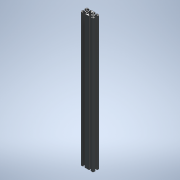
# Autodesk Inventor part: Profil_40x20_500
Saved by Autodesk Inventor 2022 (Build 260153000, 153)
## iProperties
Created: 2021-11-30
Part Number: Profil_40x20_500
Material: Generic
Document SubType Name: Modeling
Designer: Fabijan_Sven
Density: 1 g/cm^3
Appearance: Default
Author: Fabijan_Sven
Autodesk Inventor part; units mm, degrees
ref_plane "YZ Plane" through (0, 0, 0) normal (1, 0, 0) x (0, 1, 0)
ref_plane "XZ Plane" through (0, 0, 0) normal (0, 1, 0) x (-1, 0, 0)
ref_plane "XY Plane" through (0, 0, 0) normal (0, 0, 1) x (1, 0, 0)
sketch "Sketch1" plane through (0, 0, 0) normal (0, 1, 0) x (-1, 0, 0)
  line L0 (8, 10) -> (3, 10)
  line L1 (10, 3) -> (10, 8)
  line L2 (2.5, 9.5) -> (2.5, 8.2)
  line L3 (2.5, 8.2) -> (5.7198, 8.2)
  line L4 (6.0734, 7.3464) -> (3.2627, 4.5358)
  line L5 (1.8485, 3.95) -> (0, 3.95)
  line L6 (0, 3.95) -> (0, 2.15)
  line L7 (0, 2.15) -> (0, 2.15)
  line L8 (2.15, 0) -> (2.15, 0)
  line L9 (2.15, 0) -> (3.95, 0)
  line L10 (8.2, 5.7204) -> (8.2, 2.5)
  line L11 (8.2, 2.5) -> (9.5, 2.5)
  line L12 (0, 29.0836) -> (0, -4.1523) construction
  line L13 (3.95, 0) -> (3.95, 1.8491)
  line L14 (7.3464, 6.0739) -> (4.5358, 3.2633)
  arc A0 (10, 8) -> (8, 10) centre (8, 8) ccw
  arc A1 (8.2, 5.7204) -> (7.3464, 6.0739) centre (7.7, 5.7204) ccw
  arc A2 (6.0734, 7.3464) -> (5.7198, 8.2) centre (5.7198, 7.7) ccw
  arc A3 (4.5358, 3.2633) -> (3.95, 1.8491) centre (5.95, 1.8491) ccw
  arc A4 (1.8485, 3.95) -> (3.2627, 4.5358) centre (1.8485, 5.95) ccw
  arc A5 (2.15, 0) -> (0, 2.15) centre (0, 0) ccw
  arc A6 (3, 10) -> (2.5, 9.5) centre (3, 9.5) ccw
  arc A7 (9.5, 2.5) -> (10, 3) centre (9.5, 3) ccw
  line L15 (18.5462, 0) -> (-9.9601, 0) construction
  line L16 (-3, 10) -> (-8, 10)
  arc A8 (-2.5, 9.5) -> (-3, 10) centre (-3, 9.5) ccw
  line L17 (-2.5, 8.2) -> (-2.5, 9.5)
  line L18 (-5.7204, 8.2) -> (-2.5, 8.2)
  arc A9 (-5.7204, 8.2) -> (-6.0739, 7.3464) centre (-5.7204, 7.7) ccw
  line L19 (-6.0739, 7.3464) -> (-3.2633, 4.5358)
  arc A10 (-3.2633, 4.5358) -> (-1.8491, 3.95) centre (-1.8491, 5.95) ccw
  line L20 (0, 3.95) -> (-1.8491, 3.95)
  line L21 (0, 2.15) -> (0, 3.95)
  arc A11 (0, 2.15) -> (-2.15, 0) centre (0, 0) ccw
  line L22 (-3.95, 0) -> (-2.15, 0)
  line L23 (-3.95, 1.8485) -> (-3.95, 0)
  arc A12 (-3.95, 1.8485) -> (-4.5358, 3.2627) centre (-5.95, 1.8485) ccw
  line L24 (-7.3464, 6.0734) -> (-4.5358, 3.2627)
  arc A13 (-7.3464, 6.0734) -> (-8.2, 5.7198) centre (-7.7, 5.7198) ccw
  line L25 (-8.2, 2.5) -> (-8.2, 5.7198)
  line L26 (-9.5, 2.5) -> (-8.2, 2.5)
  arc A14 (-10, 3) -> (-9.5, 2.5) centre (-9.5, 3) ccw
  line L27 (-10, 8) -> (-10, 3)
  arc A15 (-8, 10) -> (-10, 8) centre (-8, 8) ccw
  line L28 (-10, -3) -> (-10, -8)
  arc A16 (-9.5, -2.5) -> (-10, -3) centre (-9.5, -3) ccw
  line L29 (-8.2, -2.5) -> (-9.5, -2.5)
  line L30 (-8.2, -5.7204) -> (-8.2, -2.5)
  arc A17 (-8.2, -5.7204) -> (-7.3464, -6.0739) centre (-7.7, -5.7204) ccw
  line L31 (-7.3464, -6.0739) -> (-4.5358, -3.2633)
  arc A18 (-4.5358, -3.2633) -> (-3.95, -1.8491) centre (-5.95, -1.8491) ccw
  line L32 (-3.95, 0) -> (-3.95, -1.8491)
  line L33 (-2.15, 0) -> (-3.95, 0)
  arc A19 (-2.15, 0) -> (0, -2.15) centre (0, 0) ccw
  line L34 (0, -3.95) -> (0, -2.15)
  line L35 (-1.8485, -3.95) -> (0, -3.95)
  arc A20 (-1.8485, -3.95) -> (-3.2627, -4.5358) centre (-1.8485, -5.95) ccw
  line L36 (-6.0734, -7.3464) -> (-3.2627, -4.5358)
  arc A21 (-6.0734, -7.3464) -> (-5.7198, -8.2) centre (-5.7198, -7.7) ccw
  line L37 (-2.5, -8.2) -> (-5.7198, -8.2)
  line L38 (-2.5, -9.5) -> (-2.5, -8.2)
  arc A22 (-3, -10) -> (-2.5, -9.5) centre (-3, -9.5) ccw
  line L39 (-8, -10) -> (-3, -10)
  arc A23 (-10, -8) -> (-8, -10) centre (-8, -8) ccw
  line L40 (3, -10) -> (8, -10)
  arc A24 (2.5, -9.5) -> (3, -10) centre (3, -9.5) ccw
  line L41 (2.5, -8.2) -> (2.5, -9.5)
  line L42 (5.7204, -8.2) -> (2.5, -8.2)
  arc A25 (5.7204, -8.2) -> (6.0739, -7.3464) centre (5.7204, -7.7) ccw
  line L43 (6.0739, -7.3464) -> (3.2633, -4.5358)
  arc A26 (3.2633, -4.5358) -> (1.8491, -3.95) centre (1.8491, -5.95) ccw
  line L44 (0, -3.95) -> (1.8491, -3.95)
  line L45 (0, -2.15) -> (0, -3.95)
  arc A27 (0, -2.15) -> (2.15, 0) centre (0, 0) ccw
  line L46 (3.95, 0) -> (2.15, 0)
  line L47 (3.95, -1.8485) -> (3.95, 0)
  arc A28 (3.95, -1.8485) -> (4.5358, -3.2627) centre (5.95, -1.8485) ccw
  line L48 (7.3464, -6.0734) -> (4.5358, -3.2627)
  arc A29 (7.3464, -6.0734) -> (8.2, -5.7198) centre (7.7, -5.7198) ccw
  line L49 (8.2, -2.5) -> (8.2, -5.7198)
  line L50 (9.5, -2.5) -> (8.2, -2.5)
  arc A30 (10, -3) -> (9.5, -2.5) centre (9.5, -3) ccw
  line L51 (10, -8) -> (10, -3)
  arc A31 (8, -10) -> (10, -8) centre (8, -8) ccw
  line L52 (-25.7204, 8.2) -> (-22.5, 8.2)
  line L53 (-22.5, 8.2) -> (-22.5, 9.5)
  arc A32 (-22.5, 9.5) -> (-23, 10) centre (-23, 9.5) ccw
  line L54 (-23, 10) -> (-28, 10)
  line L55 (-18.1515, 3.95) -> (-20, 3.95)
  line L56 (-20, 2.15) -> (-20, 2.15)
  line L57 (-17.85, 0) -> (-17.85, 0)
  line L58 (-17.85, 0) -> (-16.05, 0)
  line L59 (-11.8, 2.5) -> (-10.5, 2.5)
  line L60 (-1.4538, 0) -> (-29.9601, 0) construction
  line L61 (-16.05, 0) -> (-16.05, 1.8491)
  arc A33 (-15.4642, 3.2633) -> (-16.05, 1.8491) centre (-14.05, 1.8491) ccw
  arc A34 (-17.85, 0) -> (-20, 2.15) centre (-20, 0) ccw
  line L62 (-20, 3.95) -> (-20, 2.15)
  line L63 (-20, 3.95) -> (-21.8491, 3.95)
  arc A35 (-23.2633, 4.5358) -> (-21.8491, 3.95) centre (-21.8491, 5.95) ccw
  line L64 (-20, 2.15) -> (-20, 3.95)
  arc A36 (-20, 2.15) -> (-22.15, 0) centre (-20, 0) ccw
  arc A37 (-10.5, 2.5) -> (-10, 3) centre (-10.5, 3) ccw
  line L65 (-12.6536, -6.0734) -> (-15.4642, -3.2627)
  line L66 (-10.5, -2.5) -> (-11.8, -2.5)
  line L67 (-13.9261, -7.3464) -> (-16.7367, -4.5358)
  arc A38 (-10, -3) -> (-10.5, -2.5) centre (-10.5, -3) ccw
  line L68 (-14.2796, -8.2) -> (-17.5, -8.2)
  arc A39 (-12.6536, -6.0734) -> (-11.8, -5.7198) centre (-12.3, -5.7198) ccw
  arc A40 (-14.2796, -8.2) -> (-13.9261, -7.3464) centre (-14.2796, -7.7) ccw
  line L69 (-17, -10) -> (-12, -10)
  line L70 (-10, -8) -> (-10, -3)
  line L71 (-11.8, -2.5) -> (-11.8, -5.7198)
  arc A41 (-12, -10) -> (-10, -8) centre (-12, -8) ccw
  arc A42 (-25.7204, 8.2) -> (-26.0739, 7.3464) centre (-25.7204, 7.7) ccw
  arc A43 (-28, 10) -> (-30, 8) centre (-28, 8) ccw
  arc A44 (-27.3464, 6.0734) -> (-28.2, 5.7198) centre (-27.7, 5.7198) ccw
  line L72 (-26.0739, 7.3464) -> (-23.2633, 4.5358)
  line L73 (-27.3464, 6.0734) -> (-24.5358, 3.2627)
  arc A45 (-23.95, 1.8485) -> (-24.5358, 3.2627) centre (-25.95, 1.8485) ccw
  line L74 (-28.2, 2.5) -> (-28.2, 5.7198)
  line L75 (-30, 8) -> (-30, 3)
  line L76 (-29.5, 2.5) -> (-28.2, 2.5)
  arc A46 (-30, 3) -> (-29.5, 2.5) centre (-29.5, 3) ccw
  line L77 (-23.95, 0) -> (-22.15, 0)
  line L78 (-22.15, 0) -> (-23.95, 0)
  arc A47 (-22.15, 0) -> (-20, -2.15) centre (-20, 0) ccw
  line L79 (-23.95, 0) -> (-23.95, -1.8491)
  arc A48 (-24.5358, -3.2633) -> (-23.95, -1.8491) centre (-25.95, -1.8491) ccw
  line L80 (-21.8485, -3.95) -> (-20, -3.95)
  line L81 (-20, -3.95) -> (-20, -2.15)
  line L82 (-20, -2.15) -> (-20, -3.95)
  line L83 (-17.5, 9.5) -> (-17.5, 8.2)
  arc A49 (-18.1515, 3.95) -> (-16.7373, 4.5358) centre (-18.1515, 5.95) ccw
  arc A50 (-17, 10) -> (-17.5, 9.5) centre (-17, 9.5) ccw
  line L84 (-17.5, 8.2) -> (-14.2802, 8.2)
  line L85 (-13.9266, 7.3464) -> (-16.7373, 4.5358)
  arc A51 (-13.9266, 7.3464) -> (-14.2802, 8.2) centre (-14.2802, 7.7) ccw
  line L86 (-12.6536, 6.0739) -> (-15.4642, 3.2633)
  line L87 (-11.8, 5.7204) -> (-11.8, 2.5)
  arc A52 (-11.8, 5.7204) -> (-12.6536, 6.0739) centre (-12.3, 5.7204) ccw
  line L88 (-12, 10) -> (-17, 10)
  line L89 (-10, 3) -> (-10, 8)
  arc A53 (-10, 8) -> (-12, 10) centre (-12, 8) ccw
  line L90 (-30, -3) -> (-30, -8)
  arc A54 (-28.2, -5.7204) -> (-27.3464, -6.0739) centre (-27.7, -5.7204) ccw
  arc A55 (-30, -8) -> (-28, -10) centre (-28, -8) ccw
  line L91 (-27.3464, -6.0739) -> (-24.5358, -3.2633)
  arc A56 (-26.0734, -7.3464) -> (-25.7198, -8.2) centre (-25.7198, -7.7) ccw
  line L92 (-26.0734, -7.3464) -> (-23.2627, -4.5358)
  arc A57 (-21.8485, -3.95) -> (-23.2627, -4.5358) centre (-21.8485, -5.95) ccw
  line L93 (-28, -10) -> (-23, -10)
  line L94 (-22.5, -8.2) -> (-25.7198, -8.2)
  line L95 (-22.5, -9.5) -> (-22.5, -8.2)
  arc A58 (-23, -10) -> (-22.5, -9.5) centre (-23, -9.5) ccw
  line L96 (-20, -3.95) -> (-18.1509, -3.95)
  arc A59 (-20, -2.15) -> (-17.85, 0) centre (-20, 0) ccw
  line L97 (-16.05, -1.8485) -> (-16.05, 0)
  line L98 (-16.05, 0) -> (-17.85, 0)
  arc A60 (-16.05, -1.8485) -> (-15.4642, -3.2627) centre (-14.05, -1.8485) ccw
  arc A61 (-16.7367, -4.5358) -> (-18.1509, -3.95) centre (-18.1509, -5.95) ccw
  line L99 (-23.95, 1.8485) -> (-23.95, 0)
  line L100 (-17.5, -8.2) -> (-17.5, -9.5)
  arc A62 (-17.5, -9.5) -> (-17, -10) centre (-17, -9.5) ccw
  line L101 (-28.2, -5.7204) -> (-28.2, -2.5)
  line L102 (-28.2, -2.5) -> (-29.5, -2.5)
  arc A63 (-29.5, -2.5) -> (-30, -3) centre (-29.5, -3) ccw
  line L103 (-8, -10) -> (-12, -10)
  line L104 (-8, 10) -> (-12, 10)
  point P0 (0, 0)
  point P1 (3.95, 2.6775)
  point P2 (-2.6775, 3.95)
  point P3 (0, 0)
  point P4 (-3.95, -2.6775)
  point P5 (0, 0)
  point P6 (2.6775, -3.95)
  point P7 (0, 0)
  point P8 (-20, 0)
  point P9 (-16.05, 2.6775)
  point P10 (-20, -4.1523)
  point P11 (-22.6775, 3.95)
  point P12 (-20, 0)
  point P13 (-20, 0)
  point P14 (-20, 0)
  point P15 (-17.3225, -3.95)
  point P16 (-23.95, -2.6775)
  point P17 (-10, 3)
  dimension "d1" = 2.5
  dimension "d2" = 2.5
  dimension "d3" = 1.8
  dimension "d4" = 1.8
  dimension "d5" = 45
  dimension "d6" = 2.15
  dimension "d7" = 2.15
  dimension "d8" = 1.8
  dimension "d11" = 10
  dimension "d12" = 10
  dimension "d14" = 1.8
  dimension "d15" = 1.8
  dimension "d16" = 2.6775
  dimension "d18" = 2
  dimension "d19" = 0.5
  dimension "d20" = 2
  dimension "d21" = 2.15
  dimension "d22" = 0.5
  dimension "d25" = 360
  dimension "d31" = 20
  constraints: 210 end point, 128 point on circle, 64 centre point, 32 point on line, 16 tangent, 5 perpendicular, 5 vertical, 4 parallel, 3 equal radius, 3 horizontal, 2 coincident, 1 collinear, 420 other
  measures "d1" distance from line of point (0, 0) L2
  measures "d2" distance from line of point (0, 0) L11
  measures "d3" distance between parallel lines of L10 L1
  measures "d4" distance between parallel lines of L0 L3
  measures "d5" angle of L4 L12
  measures "d6" distance of point (0, 0) L6.end
  measures "d7" distance from line of point (0, 0) L8
  measures "d8" distance between parallel lines of L5 L7
  measures "d11" distance from line of point (0, 0) L0
  measures "d12" distance from line of point (0, 0) L1
  measures "d14" distance between parallel lines of L8 L13
  measures "d15" distance between parallel lines of L4 L14
  measures "d16" distance of L9.end point (3.95, 2.678)
  measures "d18" radius of A0
  measures "d19" radius of A1
  measures "d20" radius of A3
  measures "d21" radius of A5
  measures "d22" radius of A6
  measures "d31" distance of L17.start L52.end
extrude "Profil_40x20" add sketch "Sketch1" along normal blind 425 contours A0 L1 A7 L11 L10 A1 L14 A3 L13 L9 A5 L6 L5 A4 L4 A2 L3 L2 A6 L0 | L6 A11 L22 L23 A12 L24 A13 L25 L26 A14 L27 A15 L16 A8 L17 L18 A9 L19 A10 L20 | L47 A28 L48 A29 L49 L50 A30 L51 A31 L40 A24 L41 L42 A25 L43 A26 L44 L34 A27 L9 | A19 L34 L35 A20 L36 A21 L37 L38 A22 L39 A23 L28 A16 L29 L30 A17 L31 A18 L32 L22 | A15 A53 L104 | L27 A37 L59 L87 A52 L86 A33 L61 L58 A34 L62 L55 A49 L85 A51 L84 L83 A50 L88 A53 | L28 A41 L69 A62 L100 L68 A40 L67 A61 L96 L81 A59 L58 L97 A60 L65 A39 L71 L66 A38 | A23 L103 A41 | L62 A36 L77 L99 A45 L73 A44 L74 L76 A46 L75 A43 L54 A32 L53 L52 A42 L72 A35 L63 | L81 L80 A57 L92 A56 L94 L95 A58 L93 A55 L90 A63 L102 L101 A54 L91 A48 L79 L77 A47
body "Solid1"
